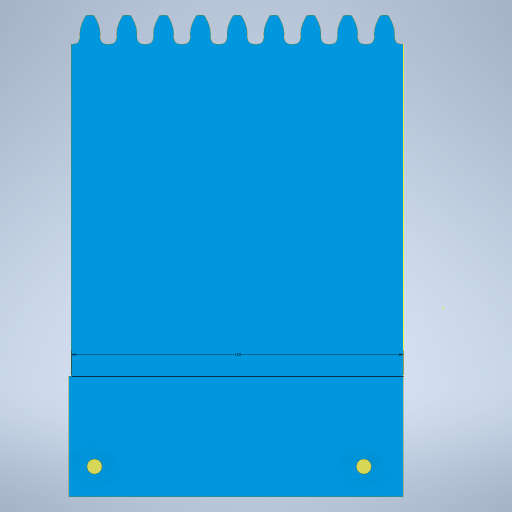
# Autodesk Inventor part: RACK_06
Saved by Autodesk Inventor 2024 (Build 280153000, 153)
## iProperties
Created: 2023-06-04
Part Number: RACK_06
Material: Generic
Document SubType Name: Modeling
Designer: Neko-san
Density: 1 g/cm^3
Appearance: Smooth - Yellow
Author: Neko-san
Autodesk Inventor part; units mm, degrees
ref_plane "YZ Plane" through (0, 0, 0) normal (1, 0, 0) x (0, 1, 0)
ref_plane "XZ Plane" through (0, 0, 0) normal (0, 1, 0) x (-1, 0, 0)
ref_plane "XY Plane" through (0, 0, 0) normal (0, 0, 1) x (1, 0, 0)
sketch "Sketch1" plane through (0, 0, 0) normal (1, 0, 0) x (0, 1, 0)
  line L0 (-13.2275, -87.5217) -> (-13.2275, 22.4783)
  line L1 (-25.7935, 22.4783) -> (-25.7935, -87.5217)
  spline S0 degree 3 poles (-25.7935, -87.5217) (-25.7583, -87.5135) (-25.6764, -87.4973) (-25.5469, -87.4814) (-25.4057, -87.4715) (-25.2643, -87.4775) (-25.1233, -87.4899) (-24.9383, -87.5272) (-24.7086, -87.5796) (-24.4775, -87.6251) (-24.2933, -87.6663) (-24.1594, -87.7123) (-24.0279, -87.7644) (-23.9028, -87.8308) (-23.7816, -87.9037) (-23.6667, -87.9864) (-23.5599, -88.0792) (-23.4573, -88.1766) (-23.3637, -88.2827) (-23.2778, -88.3951) (-23.1987, -88.5124) (-23.1035, -88.6752) (-23.0247, -88.847) (-22.9584, -89.0235) (-22.9038, -89.2039) (-22.8489, -89.4334) (-22.8087, -89.7135) (-22.7874, -89.9957) (-22.7874, -90.2786) (-22.8009, -90.5612) (-22.831, -90.8425) (-22.8607, -91.0287) (-22.8756, -91.1218) knots -0.562204 -0.562204 -0.562204 -0.562204 -0.551343 -0.537209 -0.523071 -0.508933 -0.494799 -0.48066 -0.452382 -0.424104 -0.409965 -0.395831 -0.381693 -0.367555 -0.353421 -0.339281 -0.325147 -0.311012 -0.296872 -0.282735 -0.268599 -0.254459 -0.226194 -0.212055 -0.197917 -0.169649 -0.141379 -0.113105 -0.084829 -0.056553 -0.028276 0 0 0 0
  spline S1 degree 3 poles (-22.8756, -91.1218) (-22.879, -91.1884) (-22.8858, -91.3215) (-22.8762, -91.5882) (-22.8468, -91.9203) (-22.7872, -92.316) (-22.7089, -92.7084) (-22.6141, -93.097) (-22.5049, -93.4819) (-22.3826, -93.8628) (-22.2483, -94.2396) (-22.1028, -94.6122) (-21.9469, -94.9806) (-21.7813, -95.3447) (-21.6065, -95.7045) (-21.4231, -96.06) (-21.2312, -96.411) (-21.0322, -96.758) (-20.893, -96.9854) (-20.8234, -97.0992) knots -0.639933 -0.639933 -0.639933 -0.639933 -0.619941 -0.599944 -0.559953 -0.51996 -0.479965 -0.439969 -0.399973 -0.359976 -0.319979 -0.279982 -0.239985 -0.199988 -0.15999 -0.119993 -0.079995 -0.039997 0 0 0 0
  arc A0 (-20.8234, -97.0992) -> (-18.1977, -97.0992) centre (-19.5105, -63.1245) ccw
  spline S2 degree 3 poles (-18.1977, -97.0992) (-18.1281, -96.9855) (-17.9889, -96.758) (-17.7898, -96.411) (-17.598, -96.06) (-17.4146, -95.7045) (-17.2398, -95.3447) (-17.0741, -94.9806) (-16.9183, -94.6122) (-16.7728, -94.2396) (-16.6384, -93.8628) (-16.5161, -93.4819) (-16.4069, -93.097) (-16.3122, -92.7084) (-16.2339, -92.316) (-16.1743, -91.9203) (-16.1449, -91.5882) (-16.1353, -91.3215) (-16.1421, -91.1884) (-16.1454, -91.1218) knots -0.639933 -0.639933 -0.639933 -0.639933 -0.599936 -0.559938 -0.519941 -0.479943 -0.439946 -0.399948 -0.359951 -0.319954 -0.279957 -0.239961 -0.199965 -0.159969 -0.119974 -0.07998 -0.03999 -0.019992 0 0 0 0
  spline S3 degree 3 poles (-16.1454, -91.1218) (-16.1603, -91.0287) (-16.1901, -90.8425) (-16.2202, -90.5612) (-16.2337, -90.2786) (-16.2337, -89.9957) (-16.2124, -89.7135) (-16.1721, -89.4334) (-16.1173, -89.2039) (-16.0626, -89.0235) (-15.9964, -88.847) (-15.9175, -88.6752) (-15.8224, -88.5124) (-15.7433, -88.3951) (-15.6574, -88.2827) (-15.5637, -88.1766) (-15.4611, -88.0792) (-15.3544, -87.9864) (-15.2394, -87.9037) (-15.1182, -87.8308) (-14.9932, -87.7644) (-14.8616, -87.7123) (-14.7278, -87.6663) (-14.5436, -87.6251) (-14.3125, -87.5796) (-14.0827, -87.5272) (-13.8978, -87.4899) (-13.7568, -87.4775) (-13.6154, -87.4715) (-13.4742, -87.4814) (-13.3446, -87.4973) (-13.2628, -87.5135) (-13.2275, -87.5217) knots -0.904764 -0.904764 -0.904764 -0.904764 -0.876488 -0.848211 -0.819935 -0.791659 -0.763385 -0.735115 -0.706847 -0.692709 -0.67857 -0.650305 -0.636165 -0.622029 -0.607892 -0.593752 -0.579617 -0.565483 -0.551343 -0.537209 -0.523071 -0.508933 -0.494799 -0.48066 -0.452382 -0.424104 -0.409965 -0.395831 -0.381693 -0.367555 -0.353421 -0.34256 -0.34256 -0.34256 -0.34256
  line L2 (-25.7935, 22.4783) -> (-13.2275, 22.4783)
  point P0 (-19.5105, -23.7348)
  dimension "d2" = 110
  constraints: 6 end point, 2 centre point, 2 point on circle, 1 horizontal, 16 other
  measures "d2" distance of L1.end L1.start
extrude "Extrusion1" add sketch "Sketch1" along normal blind 5
sketch "Sketch2" plane through (0, 0, 0) normal (-1, 0, 0) x (0, 0, 1)
  line L0 (-87.5217, -13.2275) -> (22.4783, -13.2275) projected
  line L1 (22.4783, -13.2275) -> (22.4783, -123.2275)
  point P0 (0, 0)
  dimension "d6" = 110
  constraints: 2 end point, 1 vertical
  measures "d6" distance of L0.end L1.end
pattern_linear "Rectangular Pattern1" count 9 spacing 12.2 along (0, -1, 0) of "Extrusion1"
sketch "Sketch3" plane through (0, -13.2275, 22.4783) normal (0, 0, 1) x (1, 0, 0)
  line L0 (0, 0) -> (5, 0) projected
  line L1 (0, -110.9171) -> (5, -110.9171)
  line L2 (5, -110.9171) -> (5, 0)
  line L3 (5, 0) -> (0, 0)
  line L4 (0, 0) -> (0, -110.9171)
  point P0 (0, 13.2275)
  constraints: 8 end point, 2 parallel, 1 horizontal, 1 perpendicular
extrude "Extrusion2" add sketch "Sketch3" along normal blind 20
sketch "Sketch4" plane through (0, 0, 0) normal (-1, 0, 0) x (0, 0, 1)
  point P0 (0, 0)
sketch "Sketch5" plane through (0, -13.2275, 42.4783) normal (0, 0, 1) x (1, 0, 0)
  line L0 (0, -110.166) -> (0, -110.9171) projected
  line L1 (0, 0) -> (5, 0) projected
  line L2 (0, -110.9171) -> (5, -110.9171)
  line L3 (5, -110.9171) -> (5, 0)
  line L4 (5, 0) -> (0, 0)
  line L5 (0, 0) -> (0, -110.9171)
  point P0 (0, 13.2275)
  point P1 (0, 0)
  point P2 (0, -110.166)
  constraints: 8 end point, 2 parallel, 1 horizontal, 1 perpendicular
extrude "Extrusion3" add sketch "Sketch5" along normal blind 20
sketch "Sketch6" plane through (0, 0, 0) normal (-1, 0, 0) x (0, 0, 1)
  line L0 (22.4783, -124.1446) -> (62.4783, -124.1446) projected
  line L1 (62.4783, -124.1446) -> (52.4783, -124.1446)
  line L2 (52.4783, -124.1446) -> (52.4783, -14.1446)
  circle A0 centre (52.4783, -115.6053) radius 2.5
  circle A1 centre (52.4783, -26.3147) radius 2.5
  point P0 (0, 0)
  dimension "d14" = 10
  dimension "d15" = 110
  dimension "d16" = 5
  dimension "d17" = 5
  constraints: 4 end point, 3 point on line, 2 centre point, 1 perpendicular
  measures "d14" distance of L0.end L1.end
  measures "d15" distance of L1.end L2.end
  measures "d16" diameter of A0
  measures "d17" diameter of A1
extrude "Extrusion4" cut sketch "Sketch6" against normal blind 20
sketch "Sketch7" plane through (5, 0, 0) normal (1, 0, 0) x (0, 0, -1)
  circle A0 centre (-52.5511, -26.317) radius 2.4987
  point P0 (0, 0)
  constraints: 1 centre point
extrude "Extrusion5" add sketch "Sketch7" along normal blind 5
sketch "Sketch8" plane through (5, 0, 0) normal (1, 0, 0) x (0, 0, -1)
  circle A0 centre (-52.4783, -115.6053) radius 2.5 projected
  circle A1 centre (-52.4783, -115.6053) radius 2.5
  point P0 (0, 0)
  constraints: 1 centre point, 1 coincident
extrude "Extrusion6" add sketch "Sketch8" along normal blind 5
sketch "Sketch9" plane through (0, 0, 0) normal (-1, 0, 0) x (0, 0, 1)
  circle A0 centre (52.4783, -115.6053) radius 2.5 projected
  circle A1 centre (52.4783, -115.6053) radius 2.5
  arc A2 (52.6381, -23.8198) -> (52.4783, -28.8147) centre (52.4783, -26.3147) ccw projected
  circle A3 centre (52.4783, -26.3147) radius 2.5
  point P0 (0, 0)
  constraints: 2 coincident, 1 centre point, 3 other
extrude "Extrusion7" add sketch "Sketch9" along normal blind 5
body "Solid1"
